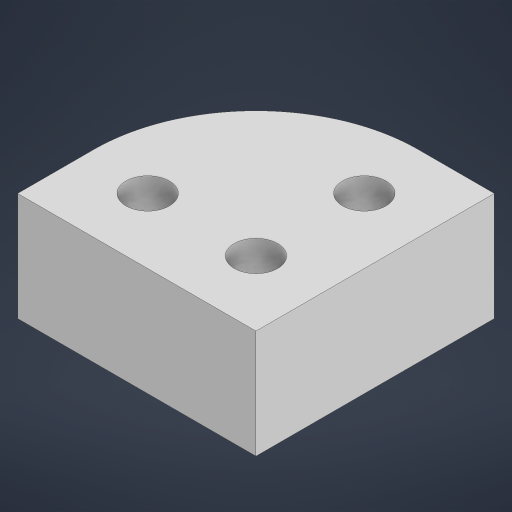
# Autodesk Inventor part: link
Saved by Autodesk Inventor 2024.3 (Build 283343000, 343)
## iProperties
Created: 2024-09-28
Part Number: link
Material: Generic
Document SubType Name: Modeling
Designer: sam
Density: 1 g/cm^3
Appearance: Default
Author: sam
Autodesk Inventor part; units mm, degrees
ref_plane "YZ Plane" through (0, 0, 0) normal (1, 0, 0) x (0, 1, 0)
ref_plane "XZ Plane" through (0, 0, 0) normal (0, 1, 0) x (-1, 0, 0)
ref_plane "XY Plane" through (0, 0, 0) normal (0, 0, 1) x (1, 0, 0)
sketch "Sketch1" plane through (0, 0, 0) normal (0, 1, 0) x (-1, 0, 0)
  line L0 (-5.5, -5.5) -> (-2, -5.5)
  line L1 (5.5, -0.5) -> (5.5, -0.5)
  line L2 (5.5, 5.5) -> (-5.5, 5.5)
  line L3 (-5.5, -0.5) -> (-5.5, -0.5)
  line L4 (-5.5, -5.5) -> (5.5, 5.5) construction
  line L5 (5.5, -5.5) -> (-5.5, 5.5) construction
  circle A0 centre (2.5, 2.5) radius 1
  circle A1 centre (-2.5, 2.5) radius 1
  line L6 (5.5, 5.5) -> (5.5, 2)
  line L7 (-5.5, 5.5) -> (-5.5, -5.5)
  circle A2 centre (-2.5, -2.5) radius 1
  arc A3 (-2, -5.5) -> (5.5, 2) centre (-2, 2) ccw
  point P0 (0, 0)
  dimension "d1" = 11
  dimension "d3" = 2
  dimension "d4" = 2
  dimension "d5" = 3
  dimension "d6" = 3
  dimension "d7" = 3
  dimension "d8" = 3
  dimension "d12" = 11
  dimension "d13" = 2
  dimension "d14" = 3
  dimension "d15" = 3
  dimension "d16" = 7.5
  constraints: 16 end point, 6 point on line, 4 centre point, 2 midpoint, 2 parallel, 2 perpendicular, 2 point on circle, 2 tangent, 1 horizontal, 1 vertical
  measures "d1" distance between parallel lines of L3 L1
  measures "d3" diameter of A0
  measures "d4" diameter of A1
  measures "d5" distance from line of L3 A1.centre
  measures "d6" distance from line of L1 A0.centre
  measures "d7" distance from line of L2 A1.centre
  measures "d8" distance from line of L2 A0.centre
  measures "d12" distance between parallel lines of L0 L2
  measures "d13" diameter of A2
  measures "d14" distance from line of L0 A2.centre
  measures "d15" distance from line of L7 A2.centre
  measures "d16" radius of A3
extrude "Extrusion1" add sketch "Sketch1" along normal blind 5
body "Solid1"
